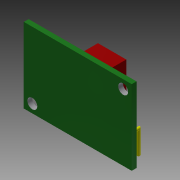
# Autodesk Inventor part: modestmard
Saved by Autodesk Inventor 2015 (Build 190159000, 159)
## iProperties
Created: 2015-02-04
Part Number: modestmard
Material: Generic
Document SubType Name: Modeling
Designer: Rafi Kurnia Putra
Density: 1 g/cm^3
Appearance: Default
Mass: 2.66687 g
Surface Area: 29.0904 cm^2
Volume: 2.66687 cm^3
Author: Rafi Kurnia Putra
Autodesk Inventor part; units mm, degrees
ref_plane "YZ Plane" through (0, 0, 0) normal (1, 0, 0) x (0, 1, 0)
ref_plane "XZ Plane" through (0, 0, 0) normal (0, 1, 0) x (-1, 0, 0)
ref_plane "XY Plane" through (0, 0, 0) normal (0, 0, 1) x (1, 0, 0)
sketch "Sketch1" plane through (0, 0, 0) normal (0, 1, 0) x (-1, 0, 0)
  line L0 (19, 13.208) -> (-19, 13.208)
  line L1 (-19, 13.208) -> (-19, -13.208)
  line L2 (-19, -13.208) -> (19, -13.208)
  line L3 (19, -13.208) -> (19, 13.208)
  line L4 (19, 13.208) -> (-19, -13.208) construction
  line L5 (-19, 13.208) -> (19, -13.208) construction
  circle A0 centre (16, -10.208) radius 1.75
  circle A1 centre (-16, 10.208) radius 1.75
  circle A2 centre (11.428, -5.518) radius 0.5
  circle A3 centre (8.888, -5.518) radius 0.5
  circle A4 centre (6.348, -5.518) radius 0.5
  circle A5 centre (3.808, -5.518) radius 0.5
  circle A6 centre (1.268, -5.518) radius 0.5
  line L6 (12.698, -6.788) -> (-0.002, -6.788)
  line L7 (-0.002, -6.788) -> (-0.002, -4.248)
  line L8 (-0.002, -4.248) -> (12.698, -4.248)
  line L9 (12.698, -4.248) -> (12.698, -6.788)
  circle A7 centre (-9.908, -5.518) radius 0.5
  circle A8 centre (-12.448, -5.518) radius 0.5
  circle A9 centre (-14.988, -5.518) radius 0.5
  line L10 (-8.638, -6.788) -> (-16.258, -6.788)
  line L11 (-16.258, -6.788) -> (-16.258, -4.248)
  line L12 (-16.258, -4.248) -> (-8.638, -4.248)
  line L13 (-8.638, -4.248) -> (-8.638, -6.788)
  line L14 (1.5071, -0.508) -> (-8.4529, -0.508)
  line L15 (-8.4529, -0.508) -> (-8.4529, 11.152)
  line L16 (-8.4529, 11.152) -> (1.5071, 11.152)
  line L17 (1.5071, 11.152) -> (1.5071, -0.508)
  point P0 (0, 0)
  dimension "d0" = 38
  dimension "d1" = 26.416
  dimension "d2" = 3.5
  dimension "d3" = 3.5
  dimension "d4" = 3
  dimension "d5" = 3
  dimension "d6" = 3
  dimension "d7" = 3
  dimension "d8" = 1
  dimension "d9" = 4.572
  dimension "d10" = 4.69
  dimension "d13" = 2.54
  dimension "d18" = 1.27
  dimension "d19" = 1.27
  dimension "d20" = 1.27
  dimension "d21" = 1.27
  dimension "d22" = 1
  dimension "d23" = 11.176
  dimension "d26" = 2.54
  dimension "d31" = 1.27
  dimension "d33" = 1.27
  dimension "d34" = 9.96
  dimension "d35" = 11.66
  dimension "d36" = 3.74
  constraints: 36 end point, 10 centre point, 8 parallel, 6 horizontal, 4 perpendicular, 2 midpoint, 1 horizontal alignment, 12 other
  measures "d0" distance of L2.end L1.end
  measures "d1" distance of L1.end L0.end
  measures "d2" diameter of A0
  measures "d3" diameter of A1
  measures "d4" distance from line of L2 A0.centre
  measures "d5" distance from line of L3 A0.centre
  measures "d6" distance from line of L1 A1.centre
  measures "d7" distance from line of L0 A1.centre
  measures "d8" diameter of A2
  measures "d9" horizontal distance of A2.centre A0.centre
  measures "d10" vertical distance of A2.centre A0.centre
  measures "d13" distance of A2.centre A3.centre
  measures "d18" distance from line of L6 A2.centre
  measures "d19" distance from line of L9 A2.centre
  measures "d20" distance from line of L8 A2.centre
  measures "d21" distance from line of L7 A6.centre
  measures "d22" diameter of A7
  measures "d23" distance of A7.centre A6.centre
  measures "d26" distance of A7.centre A8.centre
  measures "d31" distance from line of L13 A7.centre
  measures "d33" distance from line of L11 A9.centre
  measures "d34" distance of L15.end L16.end
  measures "d35" distance of L14.end L15.end
  measures "d36" distance between parallel lines of L14 L8
extrude "Extrusion1" add sketch "Sketch1" along normal blind 1.7 contours L3 L2 L1 L0
extrude "Extrusion2" add sketch "Sketch1" along normal blind 8.62 contours L14 L15 L16 L17
extrude "Extrusion3" add sketch "Sketch1" along normal blind 4.1 contours L6 L7 L8 L9 | L10 L11 L12 L13
sketch "Sketch2" plane through (19, 0, 13.208) normal (1, 0, 0) x (0, 0, -1)
  line L0 (18.9857, 6.15) -> (26.8557, 6.15)
  line L1 (0, 0) -> (26.416, 0) projected
  line L2 (18.9857, 6.15) -> (18.9857, 0)
  point P0 (13.208, 0)
  dimension "d43" = 6.15
  dimension "d44" = 7.87
  constraints: 4 end point, 1 perpendicular, 1 point on line
  measures "d43" distance of L0.start L2.end
  measures "d44" distance of L0.start L0.end
sweep "Sweep1" add profiles "Sketch1" path "Sketch2" path curves L2 L0 contours A2 | A3 | A4 | A5 | A6 | A7 | A8 | A9
sketch "Sketch3" plane through (0, 1.7, 0) normal (0, 1, 0) x (1, 0, 0)
  line L0 (-13.5449, 4.016) -> (19.3166, 4.016) construction
  line L1 (19.3166, 4.016) -> (19.3166, 0.2862) construction
  line L2 (19.3166, 0.2862) -> (-13.5449, 0.2862) construction
  line L3 (-13.5449, 0.2862) -> (-13.5449, 4.016) construction
  point P0 (0, 0)
  constraints: 2 other
body "Solid1"
